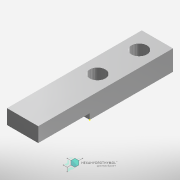
# Autodesk Inventor part: GT2 belt clamp
Saved by Autodesk Inventor 2016 (Build 200138000, 138)
## iProperties
Created: 2015-05-01
Part Number: GT2 belt clamp
Material: Aluminum 6061
Document SubType Name: Modeling
Designer: ax
Density: 2.7 g/cm^3
Appearance: Aluminum - Flat
Mass: 1.31108 g
Surface Area: 5.83079 cm^2
Volume: 0.485585 cm^3
Author: ax
Autodesk Inventor part; units mm, degrees
ref_plane "YZ Plane" through (0, 0, 0) normal (1, 0, 0) x (0, 1, 0)
ref_plane "XZ Plane" through (0, 0, 0) normal (0, 1, 0) x (-1, 0, 0)
ref_plane "XY Plane" through (0, 0, 0) normal (0, 0, 1) x (1, 0, 0)
sketch "Sketch1" plane through (0, 0, 0) normal (0, 0, 1) x (1, 0, 0)
  line L0 (0, -4.5) -> (-6, -4.5)
  line L1 (-6, -4.5) -> (-6, 11.5)
  line L2 (-6, 11.5) -> (0, 11.5)
  line L3 (0, 11.5) -> (0, -4.5)
  point P0 (0, 0)
  dimension "d0" = 6
  dimension "d1" = 16
  dimension "d17" = 0
  dimension "d18" = 11.5
  constraints: 8 end point, 2 parallel, 1 horizontal, 1 perpendicular
  measures "d0" distance of L1.end L2.end
  measures "d1" distance of L0.end L1.end
  measures "d17" distance from line of point (0, 0) L3
  measures "d18" distance from line of point (0, 0) L2
extrude "Extrusion1" add sketch "Sketch1" along normal blind 3.9
sketch "Sketch2" plane through (-6, -4.5, 0) normal (0, -1, 0) x (1, 0, 0)
  point P0 (6, 0)
sketch "Sketch3" plane through (-6, -4.5, 0) normal (0, -1, 0) x (1, 0, 0)
  line L0 (0, 3.9) -> (6, 3.9) projected
  line L1 (6, 0) -> (6, 3.9) projected
  line L2 (0, 3.9) -> (6, 3.9)
  line L3 (6, 3.9) -> (6, 1.1)
  line L4 (6, 1.1) -> (0, 1.1)
  line L5 (0, 1.1) -> (0, 3.9)
  dimension "d4" = 2.8
  constraints: 8 end point, 2 parallel, 1 horizontal, 1 perpendicular, 1 point on line
  measures "d4" distance of L2.end L3.end
extrude "Extrusion2" add sketch "Sketch3" along normal blind 9.9
sketch "Sketch4" plane through (0, 0, 3.9) normal (0, 0, 1) x (1, 0, 0)
  point P0 (0, 0)
  point P1 (-3, 8)
  point P2 (-3, 0)
hole "Hole1" at (-3, 8, 3.9) at (-3, 0, 3.9) direction (0, 0, -1) diameter 3 end through all
body "Solid1"
